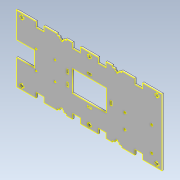
# Autodesk Inventor part: plate_2
Saved by Autodesk Inventor 2022 (Build 260153000, 153)
## iProperties
Created: 2023-04-28
Part Number: plate_2
Material: 一般
Document SubType Name: Modeling
Designer: Johnny Jou
Density: 1 g/cm^3
Appearance: 預設
Author: Johnny Jou
Autodesk Inventor part; units mm, degrees
ref_plane "YZ Plane" through (0, 0, 0) normal (1, 0, 0) x (0, 1, 0)
ref_plane "XZ Plane" through (0, 0, 0) normal (0, 1, 0) x (-1, 0, 0)
ref_plane "XY Plane" through (0, 0, 0) normal (0, 0, 1) x (1, 0, 0)
sketch "草圖1" plane through (0, 0, 0) normal (0, 0, 1) x (1, 0, 0)
  line L0 (0, 0) -> (284, 0)
  line L1 (284, 0) -> (284, -130)
  line L2 (284, -130) -> (0, -130)
  line L3 (0, -130) -> (0, 0)
  dimension "d0" = 284
  dimension "d1" = 130
  constraints: 8 end point, 2 parallel, 1 coincident, 1 horizontal, 1 perpendicular
  measures "d0" distance of L1.end L2.end
  measures "d1" distance of L0.end L1.end
extrude "擠出1" add sketch "草圖1" along normal blind 3
sketch "草圖2" plane through (0, 0, 3) normal (0, 0, 1) x (1, 0, 0)
  line L0 (35, -86.5) -> (78, -86.5)
  line L1 (78, -86.5) -> (78, -43.5)
  line L2 (78, -43.5) -> (35, -43.5)
  line L3 (35, -43.5) -> (35, -86.5)
  circle A0 centre (75, -46.5) radius 1.5
  circle A1 centre (38, -46.5) radius 1.5
  circle A2 centre (75, -83.5) radius 1.5
  circle A3 centre (38, -83.5) radius 1.5
  line L4 (0, 0) -> (0, -130) projected
  line L5 (284, 0) -> (0, 0) projected
  point P0 (74.3802, -81.4068)
  dimension "d44" = 35
  dimension "d45" = 43
  dimension "d46" = 43
  dimension "d47" = 3
  dimension "d48" = 3
  dimension "d49" = 3
  dimension "d50" = 3
  dimension "d51" = 3
  dimension "d52" = 3
  dimension "d53" = 3
  dimension "d54" = 3
  dimension "d55" = 3
  dimension "d56" = 43.5
  constraints: 8 end point, 4 centre point, 3 equal radius, 3 perpendicular
  measures "d44" distance between parallel lines of L4 L3
  measures "d45" distance of L1.end L2.end
  measures "d46" distance of L2.end L0.start
  measures "d47" distance from line of L2 A1.centre
  measures "d48" distance from line of L3 A1.centre
  measures "d49" distance from line of L2 A0.centre
  measures "d50" distance from line of L1 A0.centre
  measures "d51" distance from line of L1 A2.centre
  measures "d52" distance from line of L0 A2.centre
  measures "d53" distance from line of L3 A3.centre
  measures "d54" distance from line of L0 A3.centre
  measures "d55" diameter of A1
  measures "d56" distance between parallel lines of L5 L2
extrude "擠出2" cut sketch "草圖2" against normal up to surface (3 mm away) contours A0 | A1 | A2 | A3
sketch "草圖9" plane through (0, 0, 3) normal (0, 0, 1) x (1, 0, 0)
  line L0 (0, 0) -> (0, -130) projected
  line L1 (0, -50) -> (35, -50)
  line L2 (35, -50) -> (35, -80)
  line L3 (35, -80) -> (0, -80)
  line L4 (0, -80) -> (0, -50)
  line L5 (284, 0) -> (0, 0) projected
  point P0 (0, -80)
  dimension "d80" = 30
  dimension "d81" = 35
  dimension "d82" = 50
  constraints: 8 end point, 2 parallel, 1 horizontal, 1 perpendicular, 1 point on line
  measures "d80" distance between parallel lines of L3 L1
  measures "d81" distance between parallel lines of L0 L2
  measures "d82" distance between parallel lines of L5 L1
extrude "擠出8" cut sketch "草圖9" against normal up to surface (3 mm away)
sketch "草圖3" plane through (0, 0, 3) normal (0, 0, 1) x (1, 0, 0)
  line L0 (100.85, -42.4246) -> (100.85, -38)
  line L1 (183.15, -84.8295) -> (183.15, -92)
  line L2 (100.85, -38) -> (183.15, -38)
  line L3 (183.15, -38) -> (183.15, -92)
  line L4 (183.15, -92) -> (100.85, -92)
  line L5 (100.85, -92) -> (100.85, -38)
  line L6 (284, 0) -> (0, 0) projected
  line L7 (284, -130) -> (284, 0) projected
  line L8 (0, 0) -> (284, -130) construction
  line L9 (0, 0) -> (0, -130) projected
  line L10 (0, -130) -> (284, 0) construction
  line L11 (100.85, -38) -> (183.15, -92) construction
  line L12 (183.15, -38) -> (100.85, -92) construction
  line L13 (138, -35.05) -> (146, -35.05)
  line L14 (146, -35.05) -> (146, -38)
  line L15 (146, -38) -> (138, -38)
  line L16 (138, -38) -> (138, -35.05)
  line L17 (138, -92) -> (146, -92)
  line L18 (146, -92) -> (146, -94.95)
  line L19 (146, -94.95) -> (138, -94.95)
  line L20 (138, -94.95) -> (138, -92)
  line L21 (183.15, -61) -> (186.1, -61)
  line L22 (186.1, -61) -> (186.1, -69)
  line L23 (186.1, -69) -> (183.15, -69)
  line L24 (183.15, -69) -> (183.15, -61)
  line L25 (97.9, -50) -> (100.85, -50)
  line L26 (100.85, -50) -> (100.85, -58)
  line L27 (100.85, -58) -> (97.9, -58)
  line L28 (97.9, -58) -> (97.9, -50)
  line L29 (97.9, -72) -> (100.85, -72)
  line L30 (100.85, -72) -> (100.85, -80)
  line L31 (100.85, -80) -> (97.9, -80)
  line L32 (97.9, -80) -> (97.9, -72)
  point P0 (142, -65)
  point P1 (142, -35.05)
  point P2 (142, -65)
  point P3 (186.1, -65)
  point P4 (142, -65)
  point P5 (100.85, -80)
  point P6 (100.85, -72)
  point P7 (100.85, -58)
  point P8 (100.85, -50)
  dimension "d6" = 54
  dimension "d7" = 82.3
  dimension "d8" = 8
  dimension "d9" = 2.95
  dimension "d10" = 8
  dimension "d11" = 2.95
  dimension "d12" = 8
  dimension "d13" = 2.95
  dimension "d14" = 2.95
  dimension "d15" = 8
  dimension "d16" = 8
  dimension "d17" = 12
  dimension "d87" = 12
  constraints: 60 end point, 12 parallel, 6 horizontal, 6 midpoint, 6 perpendicular, 5 collinear, 2 point on line, 1 horizontal alignment, 1 vertical alignment
  measures "d6" distance between parallel lines of L4 L2
  measures "d7" distance between parallel lines of L5 L3
  measures "d8" distance of L18.end L19.end
  measures "d9" distance of L17.end L18.end
  measures "d10" distance of L13.start L13.end
  measures "d11" distance of L13.end L14.end
  measures "d12" distance of L21.end L22.end
  measures "d13" distance of L21.start L21.end
  measures "d14" distance of L25.start L25.end
  measures "d15" distance of L27.end L25.start
  measures "d16" distance of L31.end L29.start
  measures "d17" distance between parallel lines of L2 L25
  measures "d87" distance between parallel lines of L4 L31
extrude "擠出3" cut sketch "草圖3" against normal up to surface (3 mm away) contours L5 L27 L28 L25 | L16 L13 L14 L2 | L5 L31 L32 L29 | L21 L22 L23 L3 | L4 L18 L19 L20
sketch "草圖4" plane through (0, 0, 3) normal (0, 0, 1) x (1, 0, 0)
  line L0 (284, -130) -> (284, 0) projected
  line L1 (0, -130) -> (284, -130) projected
  circle A0 centre (211.5, -67.5) radius 2
  circle A1 centre (211.5, -96.5) radius 2
  circle A2 centre (264, -110) radius 2
  circle A3 centre (264, -62) radius 2
  point P0 (244.3247, -178.1899)
  dimension "d135" = 13.5
  dimension "d136" = 29
  dimension "d137" = 5.5
  dimension "d138" = 52.5
  dimension "d139" = 4
  dimension "d140" = 20
  dimension "d141" = 20
  constraints: 4 centre point, 3 equal radius, 2 vertical alignment
  measures "d135" vertical distance of A1.centre A2.centre
  measures "d136" distance of A0.centre A1.centre
  measures "d137" vertical distance of A3.centre A0.centre
  measures "d138" horizontal distance of A2.centre A1.centre
  measures "d139" diameter of A1
  measures "d140" distance from line of L1 A2.centre
  measures "d141" distance from line of L0 A2.centre
extrude "擠出4" cut sketch "草圖4" against normal blind 10
sketch "草圖5" plane through (0, 0, 3) normal (0, 0, 1) x (1, 0, 0)
  line L0 (79, 0) -> (97, 0)
  line L1 (97, 0) -> (97, -2.95)
  line L2 (97, -2.95) -> (79, -2.95)
  line L3 (79, -2.95) -> (79, 0)
  line L4 (187, 0) -> (205, 0)
  line L5 (205, 0) -> (205, -2.95)
  line L6 (205, -2.95) -> (187, -2.95)
  line L7 (187, -2.95) -> (187, 0)
  line L8 (187, -127.05) -> (205, -127.05)
  line L9 (205, -127.05) -> (205, -130)
  line L10 (205, -130) -> (187, -130)
  line L11 (187, -130) -> (187, -127.05)
  line L12 (79, -127.05) -> (97, -127.05)
  line L13 (97, -127.05) -> (97, -130)
  line L14 (97, -130) -> (79, -130)
  line L15 (79, -130) -> (79, -127.05)
  line L16 (284, 0) -> (0, 0) projected
  line L17 (0, -130) -> (284, -130) projected
  line L18 (0, 0) -> (0, -130) projected
  dimension "d33" = 2.95
  dimension "d34" = 18
  dimension "d36" = 2.95
  dimension "d37" = 18
  dimension "d38" = 90
  dimension "d39" = 18
  dimension "d43" = 79
  constraints: 32 end point, 9 collinear, 8 parallel, 4 horizontal, 4 perpendicular
  measures "d33" distance between parallel lines of L2 L0
  measures "d34" distance of L0.start L0.end
  measures "d36" distance between parallel lines of L14 L12
  measures "d37" distance of L13.end L14.end
  measures "d38" distance between parallel lines of L11 L13
  measures "d39" distance of L8.start L8.end
  measures "d43" distance between parallel lines of L18 L3
extrude "擠出5" cut sketch "草圖5" against normal up to surface (3 mm away)
sketch "草圖6" plane through (0, 0, 3) normal (0, 0, 1) x (1, 0, 0)
  line L0 (8.525, -3) -> (11.475, -3)
  line L1 (11.475, -3) -> (11.475, -11)
  line L2 (11.475, -11) -> (8.525, -11)
  line L3 (8.525, -11) -> (8.525, -3)
  line L4 (6, -5.525) -> (14, -5.525)
  line L5 (14, -5.525) -> (14, -8.475)
  line L6 (14, -8.475) -> (6, -8.475)
  line L7 (6, -8.475) -> (6, -5.525)
  line L8 (6, -5.525) -> (14, -8.475) construction
  line L9 (14, -5.525) -> (6, -8.475) construction
  line L10 (8.525, -11) -> (11.475, -3) construction
  line L11 (11.475, -11) -> (8.525, -3) construction
  line L12 (79, 0) -> (0, 0) construction
  line L13 (0, 0) -> (0, -130) construction
  point P0 (10, -7)
  point P1 (8.525, -8.475)
  point P2 (11.475, -8.475)
  point P3 (11.475, -5.525)
  point P4 (8.525, -5.525)
  dimension "d57" = 8
  dimension "d58" = 8
  dimension "d59" = 2.95
  dimension "d60" = 2.95
  dimension "d61" = 3
  dimension "d62" = 6
  constraints: 24 end point, 4 parallel, 2 horizontal, 2 midpoint, 2 perpendicular
  measures "d57" distance of L4.start L4.end
  measures "d58" distance of L0.end L1.end
  measures "d59" distance of L0.start L0.end
  measures "d60" distance of L4.end L5.end
  measures "d61" distance between parallel lines of L12 L0
  measures "d62" distance between parallel lines of L13 L7
extrude "擠出6" cut sketch "草圖6" against normal up to surface (3 mm away)
pattern_linear "矩形陣列1" count 2 spacing 116 along (0, -1, 0) count 3 spacing 132 along (1, 0, 0) of "擠出6"
sketch "草圖7" plane through (0, 0, 3) normal (0, 0, 1) x (1, 0, 0)
  line L0 (108.85, -44) -> (175.15, -44)
  line L1 (175.15, -44) -> (175.15, -86)
  line L2 (175.15, -86) -> (108.85, -86)
  line L3 (108.85, -86) -> (108.85, -44)
  line L4 (146, -38) -> (138, -38) projected
  line L5 (138, -92) -> (146, -92) projected
  line L6 (183.15, -69) -> (183.15, -61) projected
  line L7 (100.85, -50) -> (100.85, -58) projected
  point P0 (0, 0)
  dimension "d74" = 6
  dimension "d75" = 6
  dimension "d76" = 8
  dimension "d77" = 8
  constraints: 8 end point, 2 parallel, 1 horizontal, 1 perpendicular
  measures "d74" distance between parallel lines of L0 L4
  measures "d75" distance between parallel lines of L5 L2
  measures "d76" distance between parallel lines of L6 L1
  measures "d77" distance between parallel lines of L7 L3
extrude "擠出7" cut sketch "草圖7" against normal blind 10
sketch "草圖10" plane through (0, 0, 3) normal (0, 0, 1) x (1, 0, 0)
  line L0 (84, -5.85) -> (92, -5.85)
  line L1 (92, -5.85) -> (92, -2.95)
  line L2 (92, -2.95) -> (84, -2.95)
  line L3 (84, -2.95) -> (84, -5.85)
  line L4 (84, -5.85) -> (92, -2.95) construction
  line L5 (92, -5.85) -> (84, -2.95) construction
  line L6 (86.55, -0.4) -> (86.55, -8.4)
  line L7 (86.55, -8.4) -> (89.45, -8.4)
  line L8 (89.45, -8.4) -> (89.45, -0.4)
  line L9 (89.45, -0.4) -> (86.55, -0.4)
  line L10 (86.55, -0.4) -> (89.45, -8.4) construction
  line L11 (86.55, -8.4) -> (89.45, -0.4) construction
  line L12 (97, -2.95) -> (79, -2.95) projected
  point P0 (0, 0)
  point P1 (88, -4.4)
  point P2 (88, -4.4)
  point P3 (88, -4.4)
  point P4 (88, -2.95)
  point P5 (86.55, -2.95)
  point P6 (86.55, -5.85)
  point P7 (89.45, -5.85)
  point P8 (89.45, -2.95)
  dimension "d94" = 8
  dimension "d95" = 8
  dimension "d96" = 2.9
  dimension "d97" = 2.9
  constraints: 24 end point, 8 midpoint, 5 parallel, 2 perpendicular, 1 horizontal
  measures "d94" distance of L7.end L8.end
  measures "d95" distance of L1.end L2.end
  measures "d96" distance of L8.end L6.start
  measures "d97" distance of L0.end L1.end
extrude "擠出9" cut sketch "草圖10" against normal up to surface (3 mm away)
sketch "草圖11" plane through (0, 0, 3) normal (0, 0, 1) x (1, 0, 0)
  line L0 (109.5, 0) -> (124.5, 0)
  line L1 (124.5, 0) -> (124.5, -10)
  line L2 (124.5, -10) -> (109.5, -10)
  line L3 (109.5, -10) -> (109.5, 0)
  line L4 (109.5, 0) -> (124.5, -10) construction
  line L5 (124.5, 0) -> (109.5, -10) construction
  line L6 (159.5, 0) -> (174.5, 0)
  line L7 (174.5, 0) -> (174.5, -10)
  line L8 (174.5, -10) -> (159.5, -10)
  line L9 (159.5, -10) -> (159.5, 0)
  line L10 (159.5, 0) -> (174.5, -10) construction
  line L11 (174.5, 0) -> (159.5, -10) construction
  line L12 (187, 0) -> (97, 0) projected
  line L13 (142, 0) -> (142, -130) construction
  line L14 (97, -130) -> (187, -130) projected
  line L15 (109.5, -120) -> (124.5, -120)
  line L16 (124.5, -120) -> (124.5, -130)
  line L17 (124.5, -130) -> (109.5, -130)
  line L18 (109.5, -130) -> (109.5, -120)
  line L19 (109.5, -120) -> (124.5, -130) construction
  line L20 (124.5, -120) -> (109.5, -130) construction
  line L21 (159.5, -120) -> (174.5, -120)
  line L22 (174.5, -120) -> (174.5, -130)
  line L23 (174.5, -130) -> (159.5, -130)
  line L24 (159.5, -130) -> (159.5, -120)
  line L25 (159.5, -120) -> (174.5, -130) construction
  line L26 (174.5, -120) -> (159.5, -130) construction
  line L27 (0, -130) -> (79, -130) projected
  line L28 (79, 0) -> (0, 0) projected
  line L29 (284, 0) -> (205, 0) projected
  line L30 (205, -130) -> (284, -130) projected
  line L31 (246, -130) -> (231, -130)
  line L32 (231, -130) -> (231, -120)
  line L33 (231, -120) -> (246, -120)
  line L34 (246, -120) -> (246, -130)
  line L35 (246, -130) -> (231, -120) construction
  line L36 (231, -130) -> (246, -120) construction
  line L37 (246, -10) -> (231, -10)
  line L38 (231, -10) -> (231, 0)
  line L39 (231, 0) -> (246, 0)
  line L40 (246, 0) -> (246, -10)
  line L41 (246, -10) -> (231, 0) construction
  line L42 (231, -10) -> (246, 0) construction
  line L43 (53, -120) -> (38, -120)
  line L44 (38, -120) -> (38, -130)
  line L45 (38, -130) -> (53, -130)
  line L46 (53, -130) -> (53, -120)
  line L47 (53, -120) -> (38, -130) construction
  line L48 (38, -120) -> (53, -130) construction
  line L49 (53, -10) -> (38, -10)
  line L50 (38, -10) -> (38, 0)
  line L51 (38, 0) -> (53, 0)
  line L52 (53, 0) -> (53, -10)
  line L53 (53, -10) -> (38, 0) construction
  line L54 (38, -10) -> (53, 0) construction
  line L55 (205, -130) -> (284, -130) projected
  line L56 (0, -130) -> (79, -130) projected
  line L57 (79, 0) -> (0, 0) projected
  point P0 (117, -5)
  point P1 (167, -5)
  point P2 (117, -125)
  point P3 (167, -125)
  point P4 (238.5, -125)
  point P5 (238.5, -5)
  point P6 (45.5, -125)
  point P7 (45.5, -5)
  point P8 (38, 0)
  dimension "d100" = 25
  dimension "d101" = 25
  dimension "d102" = 15
  dimension "d103" = 15
  dimension "d104" = 10
  dimension "d105" = 10
  dimension "d106" = 25
  dimension "d107" = 25
  dimension "d108" = 10
  dimension "d109" = 10
  dimension "d110" = 15
  dimension "d111" = 15
  dimension "d116" = 15
  dimension "d117" = 15
  dimension "d118" = 15
  dimension "d119" = 15
  dimension "d120" = 71.5
  dimension "d121" = 71.5
  dimension "d122" = 71.5
  dimension "d123" = 71.5
  constraints: 98 end point, 18 midpoint, 16 parallel, 11 collinear, 8 horizontal, 8 perpendicular, 1 point on line
  measures "d100" distance from line of L13 point (167, -5)
  measures "d101" distance from line of L13 point (117, -5)
  measures "d102" distance of L0.start L0.end
  measures "d103" distance of L6.start L6.end
  measures "d104" distance of L8.end L6.start
  measures "d105" distance of L0.end L1.end
  measures "d106" distance from line of L13 point (117, -125)
  measures "d107" distance from line of L13 point (167, -125)
  measures "d108" distance of L15.end L16.end
  measures "d109" distance of L23.end L21.start
  measures "d110" distance of L15.start L15.end
  measures "d111" distance of L21.start L21.end
  measures "d116" distance of L31.start L31.end
  measures "d117" distance of L44.end L45.end
  measures "d118" distance of L37.start L37.end
  measures "d119" distance of L49.start L49.end
  measures "d120" distance of point (117, -125) point (45.5, -125)
  measures "d121" distance of point (238.5, -125) point (167, -125)
  measures "d122" distance of point (167, -5) point (238.5, -5)
  measures "d123" distance of point (45.5, -5) point (117, -5)
extrude "擠出10" cut sketch "草圖11" against normal up to surface (3 mm away)
pattern_linear "矩形陣列2" count 2 spacing 108 along (1, 0, 0) of "擠出9"
ref_plane "工作平面1" through (187, -65, 0) normal (0, -1, 0) x (1, 0, 0)
mirror "鏡射1" about plane through (187, -65, 0) normal (0, -1, 0) of "擠出9", "矩形陣列2"
sketch "草圖12" plane through (0, 0, 3) normal (0, 0, 1) x (1, 0, 0)
  line L0 (200, -124.15) -> (200, -127.05) projected
  line L1 (200, -127.05) -> (205, -127.05) projected
  line L2 (205, -127.05) -> (205, -130) projected
  line L3 (205, -130) -> (231, -130) projected
  line L4 (231, -130) -> (231, -120) projected
  line L5 (231, -120) -> (246, -120) projected
  line L6 (246, -120) -> (246, -130) projected
  line L7 (246, -130) -> (284, -130) projected
  line L8 (284, -130) -> (284, 0) projected
  line L9 (284, 0) -> (246, 0) projected
  line L10 (246, 0) -> (246, -10) projected
  line L11 (246, -10) -> (231, -10) projected
  line L12 (231, -10) -> (231, 0) projected
  line L13 (231, 0) -> (205, 0) projected
  line L14 (205, 0) -> (205, -2.95) projected
  line L15 (205, -2.95) -> (200, -2.95) projected
  line L16 (200, -2.95) -> (200, -5.85) projected
  line L17 (200, -5.85) -> (197.45, -5.85) projected
  line L18 (197.45, -5.85) -> (197.45, -8.4) projected
  line L19 (197.45, -8.4) -> (194.55, -8.4) projected
  line L20 (194.55, -8.4) -> (194.55, -5.85) projected
  line L21 (194.55, -5.85) -> (192, -5.85) projected
  line L22 (192, -5.85) -> (192, -2.95) projected
  line L23 (192, -2.95) -> (187, -2.95) projected
  line L24 (187, -2.95) -> (187, 0) projected
  line L25 (187, 0) -> (174.5, 0) projected
  line L26 (174.5, 0) -> (174.5, -10) projected
  line L27 (174.5, -10) -> (159.5, -10) projected
  line L28 (159.5, -10) -> (159.5, 0) projected
  line L29 (159.5, 0) -> (124.5, 0) projected
  line L30 (124.5, 0) -> (124.5, -10) projected
  line L31 (124.5, -10) -> (109.5, -10) projected
  line L32 (109.5, -10) -> (109.5, 0) projected
  line L33 (109.5, 0) -> (97, 0) projected
  line L34 (97, 0) -> (97, -2.95) projected
  line L35 (97, -2.95) -> (92, -2.95) projected
  line L36 (92, -2.95) -> (92, -5.85) projected
  line L37 (92, -5.85) -> (89.45, -5.85) projected
  line L38 (89.45, -5.85) -> (89.45, -8.4) projected
  line L39 (89.45, -8.4) -> (86.55, -8.4) projected
  line L40 (86.55, -8.4) -> (86.55, -5.85) projected
  line L41 (86.55, -5.85) -> (84, -5.85) projected
  line L42 (84, -5.85) -> (84, -2.95) projected
  line L43 (84, -2.95) -> (79, -2.95) projected
  line L44 (79, -2.95) -> (79, 0) projected
  line L45 (79, 0) -> (53, 0) projected
  line L46 (53, 0) -> (53, -10) projected
  line L47 (53, -10) -> (38, -10) projected
  line L48 (38, -10) -> (38, 0) projected
  line L49 (38, 0) -> (0, 0) projected
  line L50 (0, 0) -> (0, -50) projected
  line L51 (0, -50) -> (35, -50) projected
  line L52 (35, -50) -> (35, -80) projected
  line L53 (35, -80) -> (0, -80) projected
  line L54 (0, -80) -> (0, -130) projected
  line L55 (0, -130) -> (38, -130) projected
  line L56 (38, -130) -> (38, -120) projected
  line L57 (38, -120) -> (53, -120) projected
  line L58 (53, -120) -> (53, -130) projected
  line L59 (53, -130) -> (79, -130) projected
  line L60 (79, -130) -> (79, -127.05) projected
  line L61 (79, -127.05) -> (84, -127.05) projected
  line L62 (84, -127.05) -> (84, -124.15) projected
  line L63 (84, -124.15) -> (86.55, -124.15) projected
  line L64 (86.55, -124.15) -> (86.55, -121.6) projected
  line L65 (86.55, -121.6) -> (89.45, -121.6) projected
  line L66 (89.45, -121.6) -> (89.45, -124.15) projected
  line L67 (89.45, -124.15) -> (92, -124.15) projected
  line L68 (92, -124.15) -> (92, -127.05) projected
  line L69 (92, -127.05) -> (97, -127.05) projected
  line L70 (97, -127.05) -> (97, -130) projected
  line L71 (97, -130) -> (109.5, -130) projected
  line L72 (109.5, -130) -> (109.5, -120) projected
  line L73 (109.5, -120) -> (124.5, -120) projected
  line L74 (124.5, -120) -> (124.5, -130) projected
  line L75 (124.5, -130) -> (159.5, -130) projected
  line L76 (159.5, -130) -> (159.5, -120) projected
  line L77 (159.5, -120) -> (174.5, -120) projected
  line L78 (174.5, -120) -> (174.5, -130) projected
  line L79 (174.5, -130) -> (187, -130) projected
  line L80 (187, -130) -> (187, -127.05) projected
  line L81 (187, -127.05) -> (192, -127.05) projected
  line L82 (192, -127.05) -> (192, -124.15) projected
  line L83 (192, -124.15) -> (194.55, -124.15) projected
  line L84 (194.55, -124.15) -> (194.55, -121.6) projected
  line L85 (194.55, -121.6) -> (197.45, -121.6) projected
  line L86 (197.45, -121.6) -> (197.45, -124.15) projected
  line L87 (197.45, -124.15) -> (200, -124.15) projected
  line L88 (175.15, -44) -> (175.15, -86) projected
  line L89 (175.15, -86) -> (108.85, -86) projected
  line L90 (108.85, -86) -> (108.85, -44) projected
  line L91 (108.85, -44) -> (175.15, -44) projected
  line L92 (272.525, -119) -> (275.475, -119) projected
  line L93 (275.475, -119) -> (275.475, -121.525) projected
  line L94 (275.475, -121.525) -> (278, -121.525) projected
  line L95 (278, -121.525) -> (278, -124.475) projected
  line L96 (278, -124.475) -> (275.475, -124.475) projected
  line L97 (275.475, -124.475) -> (275.475, -127) projected
  line L98 (275.475, -127) -> (272.525, -127) projected
  line L99 (272.525, -127) -> (272.525, -124.475) projected
  line L100 (272.525, -124.475) -> (270, -124.475) projected
  line L101 (270, -124.475) -> (270, -121.525) projected
  line L102 (270, -121.525) -> (272.525, -121.525) projected
  line L103 (272.525, -121.525) -> (272.525, -119) projected
  line L104 (272.525, -3) -> (275.475, -3) projected
  line L105 (275.475, -3) -> (275.475, -5.525) projected
  line L106 (275.475, -5.525) -> (278, -5.525) projected
  line L107 (278, -5.525) -> (278, -8.475) projected
  line L108 (278, -8.475) -> (275.475, -8.475) projected
  line L109 (275.475, -8.475) -> (275.475, -11) projected
  line L110 (275.475, -11) -> (272.525, -11) projected
  line L111 (272.525, -11) -> (272.525, -8.475) projected
  line L112 (272.525, -8.475) -> (270, -8.475) projected
  line L113 (270, -8.475) -> (270, -5.525) projected
  line L114 (270, -5.525) -> (272.525, -5.525) projected
  line L115 (272.525, -5.525) -> (272.525, -3) projected
  line L116 (140.525, -119) -> (143.475, -119) projected
  line L117 (143.475, -119) -> (143.475, -121.525) projected
  line L118 (143.475, -121.525) -> (146, -121.525) projected
  line L119 (146, -121.525) -> (146, -124.475) projected
  line L120 (146, -124.475) -> (143.475, -124.475) projected
  line L121 (143.475, -124.475) -> (143.475, -127) projected
  line L122 (143.475, -127) -> (140.525, -127) projected
  line L123 (140.525, -127) -> (140.525, -124.475) projected
  line L124 (140.525, -124.475) -> (138, -124.475) projected
  line L125 (138, -124.475) -> (138, -121.525) projected
  line L126 (138, -121.525) -> (140.525, -121.525) projected
  line L127 (140.525, -121.525) -> (140.525, -119) projected
  line L128 (140.525, -3) -> (143.475, -3) projected
  line L129 (143.475, -3) -> (143.475, -5.525) projected
  line L130 (143.475, -5.525) -> (146, -5.525) projected
  line L131 (146, -5.525) -> (146, -8.475) projected
  line L132 (146, -8.475) -> (143.475, -8.475) projected
  line L133 (143.475, -8.475) -> (143.475, -11) projected
  line L134 (143.475, -11) -> (140.525, -11) projected
  line L135 (140.525, -11) -> (140.525, -8.475) projected
  line L136 (140.525, -8.475) -> (138, -8.475) projected
  line L137 (138, -8.475) -> (138, -5.525) projected
  line L138 (138, -5.525) -> (140.525, -5.525) projected
  line L139 (140.525, -5.525) -> (140.525, -3) projected
  line L140 (8.525, -119) -> (11.475, -119) projected
  line L141 (11.475, -119) -> (11.475, -121.525) projected
  line L142 (11.475, -121.525) -> (14, -121.525) projected
  line L143 (14, -121.525) -> (14, -124.475) projected
  line L144 (14, -124.475) -> (11.475, -124.475) projected
  line L145 (11.475, -124.475) -> (11.475, -127) projected
  line L146 (11.475, -127) -> (8.525, -127) projected
  line L147 (8.525, -127) -> (8.525, -124.475) projected
  line L148 (8.525, -124.475) -> (6, -124.475) projected
  line L149 (6, -124.475) -> (6, -121.525) projected
  line L150 (6, -121.525) -> (8.525, -121.525) projected
  line L151 (8.525, -121.525) -> (8.525, -119) projected
  line L152 (8.525, -3) -> (11.475, -3) projected
  line L153 (11.475, -3) -> (11.475, -5.525) projected
  line L154 (11.475, -5.525) -> (14, -5.525) projected
  line L155 (14, -5.525) -> (14, -8.475) projected
  line L156 (14, -8.475) -> (11.475, -8.475) projected
  line L157 (11.475, -8.475) -> (11.475, -11) projected
  line L158 (11.475, -11) -> (8.525, -11) projected
  line L159 (8.525, -11) -> (8.525, -8.475) projected
  line L160 (8.525, -8.475) -> (6, -8.475) projected
  line L161 (6, -8.475) -> (6, -5.525) projected
  line L162 (6, -5.525) -> (8.525, -5.525) projected
  line L163 (8.525, -5.525) -> (8.525, -3) projected
  circle A0 centre (264, -110) radius 2 projected
  circle A1 centre (211.5, -96.5) radius 2 projected
  circle A2 centre (211.5, -67.5) radius 2 projected
  circle A3 centre (264, -62) radius 2 projected
  line L164 (146, -92) -> (146, -94.95) projected
  line L165 (146, -94.95) -> (138, -94.95) projected
  line L166 (138, -94.95) -> (138, -92) projected
  line L167 (138, -92) -> (146, -92) projected
  line L168 (138, -38) -> (138, -35.05) projected
  line L169 (138, -35.05) -> (146, -35.05) projected
  line L170 (146, -35.05) -> (146, -38) projected
  line L171 (146, -38) -> (138, -38) projected
  line L172 (97.9, -80) -> (97.9, -72) projected
  line L173 (97.9, -72) -> (100.85, -72) projected
  line L174 (100.85, -72) -> (100.85, -80) projected
  line L175 (100.85, -80) -> (97.9, -80) projected
  line L176 (183.15, -61) -> (186.1, -61) projected
  line L177 (186.1, -61) -> (186.1, -69) projected
  line L178 (186.1, -69) -> (183.15, -69) projected
  line L179 (183.15, -69) -> (183.15, -61) projected
  line L180 (97.9, -58) -> (97.9, -50) projected
  line L181 (97.9, -50) -> (100.85, -50) projected
  line L182 (100.85, -50) -> (100.85, -58) projected
  line L183 (100.85, -58) -> (97.9, -58) projected
  circle A4 centre (75, -83.5) radius 1.5 projected
  circle A5 centre (38, -46.5) radius 1.5 projected
  circle A6 centre (38, -83.5) radius 1.5 projected
  circle A7 centre (75, -46.5) radius 1.5 projected
